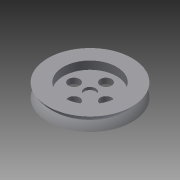
# Autodesk Inventor part: StringWheel
Saved by Autodesk Inventor 2015 (Build 190159000, 159)
## iProperties
Created: 2016-02-18
Part Number: StringWheel
Material: Generic
Document SubType Name: Modeling
Designer: Hatch
Density: 1 g/cm^3
Appearance: Default
Author: Hatch
Autodesk Inventor part; units mm, degrees
ref_plane "YZ Plane" through (0, 0, 0) normal (1, 0, 0) x (0, 1, 0)
ref_plane "XZ Plane" through (0, 0, 0) normal (0, 1, 0) x (-1, 0, 0)
ref_plane "XY Plane" through (0, 0, 0) normal (0, 0, 1) x (1, 0, 0)
sketch "Sketch1" plane through (0, 0, 0) normal (0, 1, 0) x (-1, 0, 0)
  circle A0 centre (0, 0) radius 17.5
  dimension "d0" = 35
  constraints: 1 centre point, 1 coincident
  measures "d0" diameter of A0
extrude "Extrusion1" add sketch "Sketch1" along normal blind 5
sketch "Sketch2" plane through (0, 5, 0) normal (0, 1, 0) x (1, 0, 0)
  circle A0 centre (0, 0) radius 10
  dimension "d3" = 20
  constraints: 1 centre point, 1 coincident
  measures "d3" diameter of A0
extrude "Extrusion2" cut sketch "Sketch2" against normal blind 3
sketch "Sketch3" plane through (0, 2, 0) normal (0, 1, 0) x (1, 0, 0)
  circle A0 centre (-6, 0) radius 2.125
  circle A1 centre (-6, 0) radius 2.125
  point P0 (0, 0)
  dimension "d7" = 4.25
  constraints: 2 centre point, 1 coincident, 1 concentric
  measures "d7" diameter of A0
extrude "Extrusion3" cut sketch "Sketch3" against normal through all
pattern_circular "Circular Pattern1" count 4 over 360 about axis through (0, 5, 0) along (0, -1, 0) of "Extrusion3"
sketch "Sketch4" plane through (0, 2, 0) normal (0, 1, 0) x (1, 0, 0)
  circle A0 centre (0, 0) radius 2.125
  dimension "d13" = 4.25
  constraints: 1 centre point, 1 coincident
  measures "d13" diameter of A0
extrude "Extrusion4" cut sketch "Sketch4" against normal blind 1
sketch "Sketch5" plane through (0, 5, 0) normal (0, 1, 0) x (1, 0, 0)
  circle A0 centre (0, 0) radius 10 projected
  circle A1 centre (0, 0) radius 17.5 projected
  circle A2 centre (0, 0) radius 2.125 projected
  circle A3 centre (0, 0) radius 13.75
  circle A4 centre (0, 0) radius 17.5
  constraints: 2 centre point, 2 coincident
extrude "Extrusion5" cut sketch "Sketch5" against normal through all contours A1
sketch "Sketch6" plane through (0, 5, 0) normal (0, 1, 0) x (1, 0, 0)
  circle A0 centre (0, 0) radius 13.75
  circle A1 centre (0, 0) radius 15.75
  dimension "d18" = 31.5
  constraints: 2 centre point, 2 coincident
  measures "d18" diameter of A1
sketch "Sketch7" plane through (0, 0, 0) normal (0, -1, 0) x (1, 0, 0)
  circle A0 centre (0, 0) radius 2.125 projected
  circle A1 centre (0, 0) radius 13.75
  circle A2 centre (0, 0) radius 15.75
  dimension "d19" = 31.5
  constraints: 2 centre point, 2 coincident
  measures "d19" diameter of A2
extrude "Extrusion6" add sketch "Sketch6" against normal blind 2.5
fillet "Fillet1" radius 9 1 edges at (-15.75, 2.5, 0)
extrude "Extrusion7" add sketch "Sketch7" against normal blind 2.5 contours A2
fillet "Fillet2" radius 9 1 edges at (-15.75, 2.5, 0)
body "Solid1"
